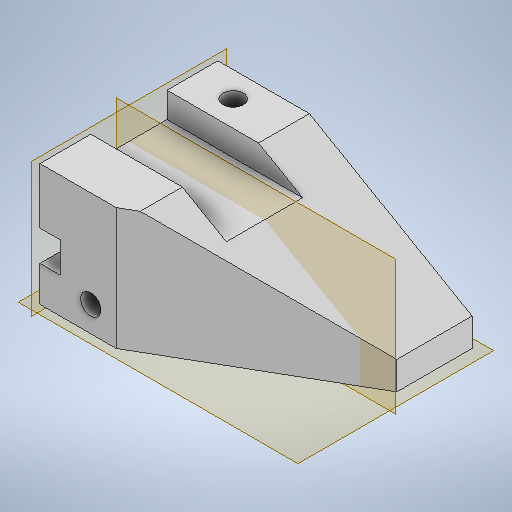
# Autodesk Inventor part: chap3ex3
Saved by Autodesk Inventor 2025.2 (Build 292293000, 293)
## iProperties
Created: 2025-02-01
Part Number: chap3ex3
Material: Generic
Document SubType Name: Modeling
Designer: Moofin
Density: 1 g/cm^3
Appearance: Default
Author: Moofin
Autodesk Inventor part; units mm, degrees
sketch "Sketch2" plane through (0, 0, 0) normal (0, 1, 0) x (-1, 0, 0)
  line L0 (0, -87.5) -> (-250, -87.5)
  line L1 (-250, -87.5) -> (-250, 87.5)
  line L2 (-250, 87.5) -> (0, 87.5)
  line L3 (0, 87.5) -> (0, -87.5)
  line L4 (0, -122.5) -> (0, 122.5) projected
  line L5 (-300, 0) -> (50, 0) projected
  point P0 (0, 0)
  dimension "d0" = 0
  dimension "d1" = 250
  dimension "d2" = 175
  dimension "d3" = 87.5
  constraints: 8 end point, 2 parallel, 1 horizontal, 1 perpendicular
  measures "d0" distance between parallel lines of L4 L3
  measures "d1" distance between parallel lines of L1 L3
  measures "d2" distance between parallel lines of L0 L2
  measures "d3" distance between parallel lines of L5 L0
extrude "Extrusion1" add sketch "Sketch2" along normal blind 120
chamfer "Chamfer1" distance 175 angle 30 1 edges at (250, 60, 87.5) measured on face at (83.3333, 40, 87.5)
chamfer "Chamfer2" distance 160 angle 30 1 edges at (250, 120, -50.5181) measured on face at (108.3333, 120, -4.5121)
sketch "Sketch4" plane through (0, 0, 87.5) normal (0, 0, 1) x (1, 0, 0)
  line L0 (0, 65) -> (20, 65)
  line L1 (20, 65) -> (20, 35)
  line L2 (20, 35) -> (0, 35)
  line L3 (0, 35) -> (0, 65)
  line L4 (0, 144) -> (0, -24) projected
  line L5 (-50, 0) -> (300, 0) projected
  point P0 (0, 0)
  dimension "d15" = 0
  dimension "d16" = 30
  dimension "d17" = 20
  dimension "d18" = 35
  constraints: 8 end point, 2 parallel, 1 horizontal, 1 perpendicular
  measures "d15" distance between parallel lines of L4 L3
  measures "d16" distance between parallel lines of L2 L0
  measures "d17" distance between parallel lines of L1 L3
  measures "d18" distance between parallel lines of L5 L2
sketch "Sketch6" plane through (0, 0, 87.5) normal (0, 0, 1) x (1, 0, 0)
  circle A0 centre (50, 25) radius 10
  line L0 (-50, 0) -> (300, 0) projected
  line L1 (0, 144) -> (0, -24) projected
  point P0 (0, 0)
  dimension "d23" = 20
  dimension "d24" = 25
  dimension "d25" = 50
  constraints: 1 centre point
  measures "d23" diameter of A0
  measures "d24" distance from line of L0 A0.centre
  measures "d25" distance from line of L1 A0.centre
sketch "Sketch7" plane through (250, 0, -87.5) normal (0, 0, -1) x (-1, 0, 0)
  line L0 (230, 35) -> (250, 35) projected
  line L1 (250, 65) -> (230, 65) projected
  line L2 (230, 65) -> (230, 35) projected
  point P0 (250, 0)
extrude "Extrusion3" cut sketch "Sketch4" against normal up to next
extrude "Extrusion4" cut sketch "Sketch6" against normal up to surface (175 mm away)
sketch "Sketch8" plane through (0, 120, 0) normal (0, 1, 0) x (1, 0, 0)
  circle A0 centre (40, 62.5) radius 10
  line L0 (90, 87.5) -> (0, 87.5) projected
  line L1 (0, 87.5) -> (0, -87.5) projected
  point P0 (0, 0)
  dimension "d28" = 20
  dimension "d29" = 25
  dimension "d30" = 40
  constraints: 1 centre point
  measures "d28" diameter of A0
  measures "d29" distance from line of L0 A0.centre
  measures "d30" distance from line of L1 A0.centre
extrude "Extrusion5" cut sketch "Sketch8" against normal up to surface (120 mm away)
sketch "Sketch9" plane through (0, 120, 0) normal (0, 1, 0) x (1, 0, 0)
  line L0 (0, 37.5) -> (250, 37.5)
  line L1 (250, 37.5) -> (250, -37.5)
  line L2 (250, -37.5) -> (0, -37.5)
  line L3 (0, -37.5) -> (0, 37.5)
  line L4 (90, 87.5) -> (0, 87.5) projected
  line L5 (0, 87.5) -> (0, -87.5) projected
  point P0 (0, 0)
  dimension "d33" = 50
  dimension "d34" = 75
  dimension "d35" = 0
  dimension "d36" = 250
  constraints: 8 end point, 2 parallel, 1 horizontal, 1 perpendicular
  measures "d33" distance between parallel lines of L4 L0
  measures "d34" distance between parallel lines of L2 L0
  measures "d35" distance between parallel lines of L5 L3
  measures "d36" distance between parallel lines of L3 L1
extrude "Extrusion6" cut sketch "Sketch9" against normal blind 25
equation "\"d3\" = 0.5 * d2"
body "Solid1"
